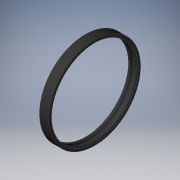
# Autodesk Inventor part: SKF_W 61810-2RS1_PART2
Saved by Autodesk Inventor 2019 (Build 230136000, 136)
## iProperties
Created: 2022-09-01
Part Number: SKF_W 61810-2RS1_PART2
Material: Generic
Catalog Web Link: www.cadenas.de
Description: -Deep groove ball bearings
Vendor: SKF
Document SubType Name: Modeling
Designer: psAdmin
Manufacturer: SKF
Mass: 51 g
Surface Area: 37.4059 cm^2
Volume: 2.87296 cm^3
Density: 1 g/cm^3
Appearance: PSOLRGB-175-175-175
Category: PARTsolutions
Company: SKF
Title: SKF_W 61810-2RS1_PART2
Author: Cadenas PARTsolutions
Comments: Deep groove ball bearings
PSOL_IDENT_0: {$CADENAS_DATA/23d-libs/skf/bearings_units_and_housings/ball_bearings/deep_groove_ball_bearings/bb1_
PSOL_IDENT_1: 001_101.prj},211 {VTYP=3D},{NB=SKF_W 61810-2RS1_PART2},{LINA=SKF_W 61810-2RS1_PART2},{NN=BB1_001_101
PSOL_IDENT_2: _PART2},{NOPRJ=TRUE},{DATE=04.08.2022 15:25:15},{GEOMDATE=04.07.2022 10:54:51},{VERSION=},{LINEID=19
PSOL_IDENT_3: 000},{WBVAR=},{WBNUMERIC=}  {NB=SKF_W 61810-2RS1_PART2},{LINA=SKF_W 61810-2RS1_PART2},{KT=DUMMY},{DE
PSOL_IDENT_4: SIGNATION=W 61810-2RS1},{R12=0.30},{DD=50.000},{D=65.000},{B=7.000},{C=},{CX=},{CXX=},{CA=0.000},{XX
PSOL_IDENT_5: VARIANT=},{XXDESIGN=Single row stainless steel},{XXSEALING=Contact seal on both sides},{DESIGN=dgbbw
PSOL_IDENT_6: 2rs},{DESIGNIR=dgbbw2rs},{VARIANT=},{DD1=54.67},{DD2=54.67},{DD2X=},{DD2A=54.67},{D1=60.30},{D1X=0.0
PSOL_IDENT_7: 0},{D2=61.55},{D2A=61.55},{D3=},{D3X=},{D3A=0.000},{D4=},{HH=0.000},{BB=0.000},{BBX=},{BBA=0.000},{F
PSOL_IDENT_8: F=},{R0MAX=0.000},{R0=0.000},{PITCH=57.50},{DW=3.969},{DDAMIN=52.000},{DDAMAX=54.500},{DDBMIN=0.000}
PSOL_IDENT_9: ,{DDBMAX=0.000},{DBMIN=0.000},{DAMAX=63.000},{BBAMIN=0.000},{CAMAX=0.000},{RAMAX=0.300},{LOAD1=5.070
PSOL_IDENT_10: },{LOAD2=5.500},{LOAD3=0.236},{SPEED1=0},{SPEED2=6000},{KR=0.020},{F0=15.300},{Z=23},{II=1},{MASS=0.
PSOL_IDENT_11: 051},{BEARING=W 61810-2RS1},{RING=},{HELP=2.350},{HELP2=1.725},{DD1ALG=27.335},{YALG=27.335},{PITCH1=
PSOL_IDENT_12: 57.500},{DW1=3.969},{YALG1=30.150},{HALG1=2.350},{SH=27.335},{CU=0.606},{HALG=2.335},{B1=0},{SHIELDH
PSOL_IDENT_13: ELP=2},{D4A=0.000},{FFA=0.000},{RS1=},{HELP3=0}
NB: SKF_W 61810-2RS1_PART2
NT: Deep groove ball bearings
NBSYN: SKF_$DESIGNATION._PART2
LINA: SKF_W 61810-2RS1_PART2
CATALOG: SKF
DESIGNATION: W 61810-2RS1
R12: 0.3
DD: 50
D: 65
B: 7
XXDESIGN: Single row stainless steel
XXSEALING: Contact seal on both sides
DD2: 54.67
D2: 61.55
LOAD1: 5.07
LOAD2: 5.5
LOAD3: 0.236
SPEED1: 0
SPEED2: 6000
BEARING: W 61810-2RS1
SUPPLIER: SKF
ARTICLENO: SKF_W 61810-2RS1_PART2
BOMINFO: SKF_W 61810-2RS1_PART2
CREATOR: CADENAS GmbH
Autodesk Inventor part; units mm, degrees
ref_plane "YZ Plane" through (0, 0, 0) normal (1, 0, 0) x (0, 1, 0)
ref_plane "XZ Plane" through (0, 0, 0) normal (0, 1, 0) x (-1, 0, 0)
ref_plane "XY Plane" through (0, 0, 0) normal (0, 0, 1) x (1, 0, 0)
sketch "Sketch_16" plane through (0, 0, 0) normal (0, 0, 1) x (1, 0, 0)
  line L0 (50, 0) -> (-50, 0)
  line L1 (0, 30.775) -> (0.09, 30.775)
  arc A0 (0.45, 30.775) -> (0.09, 30.775) centre (0.27, 30.775) ccw
  line L2 (0.45, 30.775) -> (0.5602, 30.15)
  line L3 (0.5602, 30.15) -> (2.0935, 30.15)
  arc A1 (4.9065, 30.15) -> (2.0935, 30.15) centre (3.5, 28.75) ccw
  line L4 (4.9065, 30.15) -> (6.4398, 30.15)
  line L5 (6.4398, 30.15) -> (6.55, 30.775)
  arc A2 (6.91, 30.775) -> (6.55, 30.775) centre (6.73, 30.775) ccw
  line L6 (6.91, 30.775) -> (7, 30.775)
  line L7 (7, 30.775) -> (7, 32.2)
  arc A3 (7, 32.2) -> (6.7, 32.5) centre (6.7, 32.2) ccw
  line L8 (6.7, 32.5) -> (0.3, 32.5)
  arc A4 (0.3, 32.5) -> (0, 32.2) centre (0.3, 32.2) ccw
  line L9 (0, 32.2) -> (0, 30.775)
  constraints: 20 end point, 10 point on circle, 5 centre point
revolve "Revolution1" add sketch "Sketch_16" angle 360 about axis through (50, 0, 0) along (1, 0, 0)
body "Solid1"
